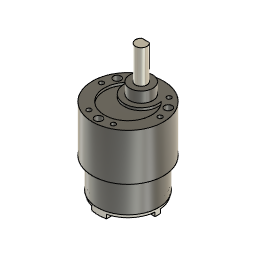
Gearbox Motor (Autodesk Fusion 360 design; units mm, degrees)
Autodesk Fusion 360 part; units mm, degrees
sketch "Sketch1" plane through (0, 0, 0) normal (0, 0, 1) x (1, 0, 0) in component "Body Upper"
  circle A0 centre (0, 0) radius 18.35
  circle A1 centre (0, 6.85) radius 6
  line L0 (0, 18.35) -> (0, -18.35) construction
  circle A2 centre (0, 6.85) radius 8.8
  circle A3 centre (0, 0) radius 12.2
  line L1 (0, -18.35) -> (0, -12.2) construction
  circle A4 centre (0, -15.275) radius 1.95
  circle A5 centre (0, 0) radius 15.275 construction
  circle A6 centre (6.3512, -13.892) radius 1.15
  circle A7 centre (-6.3512, -13.892) radius 1.15
  circle A8 centre (0, 6.85) radius 3
  dimension "d1" = 36.7
  dimension "d3" = 12
  dimension "d4" = 25.2
  dimension "d5" = 2.8
  dimension "d6" = 6.15
  dimension "d7" = 3.9
  dimension "d8" = 2.3
  dimension "d9" = 6.5
  dimension "d15" = 6
  constraint coincident A0.centre A3.centre
  constraint coincident A0 L0.start
  constraint coincident A0 L0.end
  constraint vertical L0
  constraint coincident A1.centre L0
  constraint coincident L0 L1.end
  constraint coincident A3 L1.end
  constraint midpoint L1 A4.centre
  constraint concentric A0 A5
  constraint coincident A4.centre A5
  constraint coincident A5 A6.centre
  constraint symmetric L0 A6 A7
  constraint concentric A1 A8
  measures "d1" diameter of A0
  measures "d3" diameter of A1
  measures "d4" distance of A1.centre L0.end
  measures "d7" diameter of A4
  measures "d8" diameter of A6
  measures "d9" distance of A4.centre A6.centre
  measures "d15" diameter of A8
extrude "Extrude1" add sketch "Sketch1" along normal blind 24.2 contours A0 | A1 A3 | A1 A2 A3 | A1 A3 | A1 A2 A3 | A2 A3 | A4 | A6 | A7 | A8 makes body 1 in component "Body Upper"
extrude "Extrude2" cut sketch "Sketch1" against normal blind 1.3 from surface at 24.2 contours A2 A3 bodies 1 in component "Body Upper"
extrude "Extrude3" add sketch "Sketch1" along normal blind 5.5 from surface at 24.2 contours A1 A3 | A1 A3 bodies 1 in component "Body Upper"
extrude "Extrude4" cut sketch "Sketch1" against normal blind 4 from surface at 24.2 contours A4 | A6 | A7 bodies 1 in component "Body Upper"
pattern_circular "C-Pattern1" count 3 over 360 about axis through (0, 0, 1.75) along (0, 0, 1) of "Extrude4" in component "Body Upper"
sketch "Sketch1 (2)" plane through (0, 0, 0) normal (0, 0, 1) x (1, 0, 0) in component "Body Lower"
  circle A0 centre (0, 0) radius 15.9
  circle A1 centre (0, 0) radius 15.45
  circle A2 centre (0, 0) radius 14.2
  line L0 (0, -23) -> (0, -26) construction
  line L1 (28, 0) -> (32, 0) construction
  circle A3 centre (0, 0) radius 3.6
  line L2 (-3.85, -14.9626) -> (-3.85, -3.0704)
  line L3 (-3.85, 3.0704) -> (-3.85, 14.9626)
  line L4 (-15.3818, 1.45) -> (-4.7061, 1.45)
  line L5 (-15.3818, -1.45) -> (-4.7061, -1.45)
  line L6 (4.7061, -1.45) -> (15.3818, -1.45)
  line L7 (3.85, -14.9626) -> (3.85, -3.0704)
  line L8 (3.85, 3.0704) -> (3.85, 14.9626)
  line L9 (4.7061, 1.45) -> (15.3818, 1.45)
  arc A4 (4.7061, 1.45) -> (3.85, 3.0704) centre (0, 0) ccw
  arc A5 (3.85, -3.0704) -> (4.7061, -1.45) centre (0, 0) ccw
  arc A6 (-3.85, 3.0704) -> (-4.7061, 1.45) centre (0, 0) ccw
  arc A7 (-4.7061, -1.45) -> (-3.85, -3.0704) centre (0, 0) ccw
  dimension "d24" = 31.8
  dimension "d25" = 0.45
  dimension "d28" = 1.7
  dimension "d29" = 7.7
  dimension "d30" = 2.9
  dimension "d31" = 7.2
  constraint coincident A0.centre A1.centre
  constraint coincident A1 L7.start
  constraint coincident A1 L8.end
  constraint vertical L7
  constraint parallel L0 L7
  constraint symmetric L7.start L0 L2.start
  constraint symmetric L8.end L0 L3.end
  constraint horizontal L1
  constraint coincident A1 L4.start
  constraint horizontal L4
  constraint symmetric L1 L4.start L5.start
  constraint concentric A3 A6
  constraint collinear L2 L3
  constraint coincident L5.end A6
  constraint coincident L7.end A6
  constraint collinear L7 L8
  constraint coincident L9.start A6
  constraint concentric A4 A6
  constraint concentric A5 A6
  constraint concentric A6 A7
  constraint coincident A1 L9.end
  constraint coincident A1 L6.end
  measures "d24" diameter of A0
  measures "d29" distance of L2 L7
  measures "d30" distance of L4 L5
  measures "d31" diameter of A3
extrude "Extrude1'" add sketch "Sketch1 (2)" against normal blind 15.4 separate body contours A0 makes body 2 in component "Body Lower"
extrude "Extrude2'" add sketch "Sketch1 (2)" along normal blind 2 from surface at -14.2 separate body contours A1 A2 L6 L9 | A1 A2 L8 L9 | A1 A2 L6 L7 | A1 A2 L3 L8 | A2 L8 L9 A4 | A2 L2 L3 L4 L5 L6 L7 L8 L9 A4 A5 A6 A7 | A1 A2 L2 L7 | A2 L6 L7 A5 | A1 A2 L3 L4 | A1 A2 L2 L5 | A1 A2 L4 L5 | A2 L3 L4 A6 | A2 L2 L5 A7 | A3 makes body 3 in component "Body Lower"
extrude "Extrude3'" add sketch "Sketch1 (2)" against normal blind 2.8 from surface at -14.2 contours A1 A2 L6 L9 | A1 A2 L8 L9 | A1 A2 L6 L7 | A1 A2 L3 L8 | A1 A2 L2 L7 | A1 A2 L3 L4 | A1 A2 L2 L5 | A1 A2 L4 L5 bodies 3 in component "Body Lower"
extrude "Extrude4'" add sketch "Sketch1 (2)" against normal blind 4.8 from surface at -14.2 contours A1 A2 L6 L9 | A1 A2 L3 L8 | A2 L2 L3 L4 L5 L6 L7 L8 L9 A4 A5 A6 A7 | A1 A2 L2 L7 | A1 A2 L4 L5 | A3 bodies 3 in component "Body Lower"
extrude "Extrude5" add sketch "Sketch1 (2)" against normal blind 3.35 from surface at -19 contours A3 bodies 3 in component "Body Lower"
sketch "Sketch1 (3)" plane through (0, 0, 0) normal (0, 0, 1) x (1, 0, 0) in component "Rod"
  circle A0 centre (0, 6.85) radius 3
  line L0 (-1.9261, 9.15) -> (1.9261, 9.15)
  point P0 (0, 9.85)
  dimension "d44" = 0.7
  constraint coincident A0 L0.start
  constraint coincident A0 L0.end
  constraint coincident A0 P0
  measures "d44" distance of L0 P0
extrude "Extrude1''" add sketch "Sketch1 (3)" along normal blind 10.8 from surface at 24.2 separate body makes body 4 in component "Rod"
extrude "Extrude2''" add sketch "Sketch1 (3)" along normal blind 12 from surface at 35 contours A0 L0 picked at (-0.4913, 7.3063) bodies 4 in component "Rod"
component "Rod" placed x (1, 0, 0) y (0, 1, 0) z (0, 0, 1) at (0, 0, 0)
component "Body Upper" placed x (1, 0, 0) y (0, 1, 0) z (0, 0, 1) at (0, 0, 0)
component "Body Lower" placed x (1, 0, 0) y (0, 1, 0) z (0, 0, 1) at (0, 0, 0)
equation "d28 = 1.25 mm + 0.45 mm"
equation "d32 = -2.8 mm + 1.6 mm"
equation "d46 = 5.5 mm + 5.3 mm"
